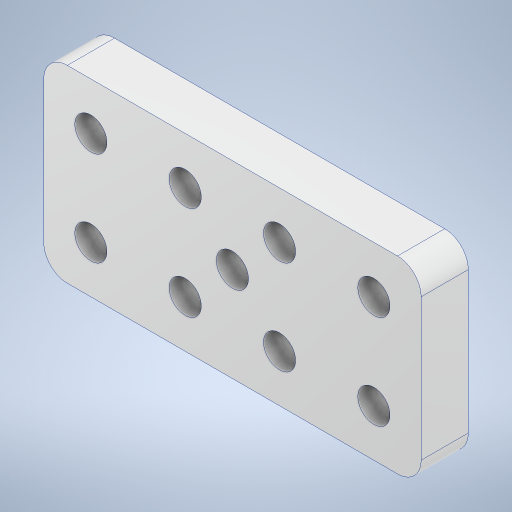
# Autodesk Inventor part: IntakeShoulder
Saved by Autodesk Inventor 2023 (Build 270158000, 158)
## iProperties
Created: 2022-11-06
Part Number: IntakeShoulder
Material: Aluminum 6061
Document SubType Name: Modeling
Designer: zac-h
Density: 2.7 g/cm^3
Appearance: Aluminum - Flat
Mass: 11.2632 g
Surface Area: 43.63 cm^2
Volume: 4.17154 cm^3
Author: zac-h
Autodesk Inventor part; units mm, degrees
ref_plane "YZ Plane" through (0, 0, 0) normal (1, 0, 0) x (0, 1, 0)
ref_plane "XZ Plane" through (0, 0, 0) normal (0, 1, 0) x (-1, 0, 0)
ref_plane "XY Plane" through (0, 0, 0) normal (0, 0, 1) x (1, 0, 0)
sketch "Sketch1" plane through (0, 0, 0) normal (0, 0, 1) x (1, 0, 0)
  circle A0 centre (0, 0) radius 2.159
  line L0 (0, 0) -> (38.1, 0) construction
  line L1 (0, 0) -> (0, 12.7) construction
  circle A1 centre (12.7, 0) radius 2.159
  circle A2 centre (25.4, 0) radius 2.159
  circle A3 centre (38.1, 0) radius 2.159
  circle A4 centre (0, 12.7) radius 2.159
  circle A5 centre (12.7, 12.7) radius 2.159
  circle A6 centre (25.4, 12.7) radius 2.159
  circle A7 centre (38.1, 12.7) radius 2.159
  circle A8 centre (19.05, 6.35) radius 2.159
  line L2 (12.7, 12.7) -> (25.4, 0) construction
  line L3 (-6.35, 19.05) -> (44.45, 19.05)
  line L4 (44.45, 19.05) -> (44.45, -6.35)
  line L5 (44.45, -6.35) -> (-6.35, -6.35)
  line L6 (-6.35, -6.35) -> (-6.35, 19.05)
  circle A9 centre (0, 12.7) radius 6.35 construction
  circle A10 centre (38.1, 0) radius 6.35 construction
  dimension "d0" = 4.318
  dimension "d1" = 38.1
  dimension "d9" = 12.7
  dimension "d12" = 12.7
  dimension "d15" = 12.7
  dimension "d18" = 4.318
  dimension "d19" = 25.4
  constraints: 14 end point, 11 centre point, 4 tangent, 3 coincident, 3 horizontal, 2 parallel, 2 vertical, 1 equal radius, 1 midpoint, 1 perpendicular, 14 other
  measures "d0" diameter of A0
  measures "d1" distance of L0.start L0.end
  measures "d9" distance of L0.start L1.end
  measures "d12" distance of L0.start A1.centre
  measures "d15" distance of L0.start A4.centre
  measures "d18" diameter of A8
  measures "d19" distance of L3.end L4.end
extrude "Extrusion1" add sketch "Sketch1" along normal blind 6.35
fillet "Fillet1" radius 3.175 4 edges at (44.45, 19.05, 3.175) (44.45, -6.35, 3.175) (-6.35, -6.35, 3.175) (-6.35, 19.05, 3.175)
body "Solid1"
